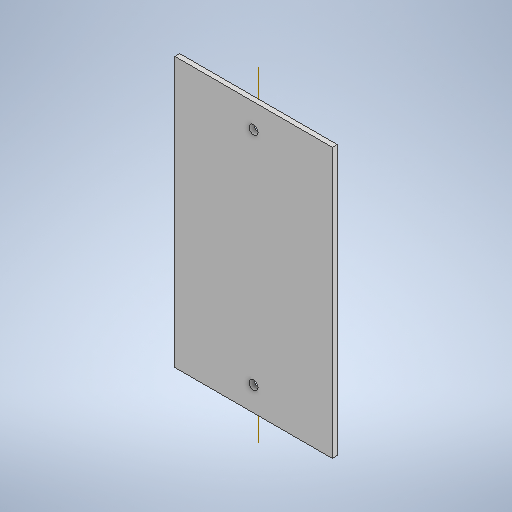
# Autodesk Inventor part: 빵판
Saved by Autodesk Inventor 2025 (Build 290162000, 162)
## iProperties
Created: 2024-06-01
Part Number: 빵판
Material: 일반
Document SubType Name: Modeling
Designer: ckhye
Density: 1 g/cm^3
Appearance: 기본값
Author: ckhye
Autodesk Inventor part; units mm, degrees
ref_plane "YZ Plane" through (0, 0, 0) normal (1, 0, 0) x (0, 1, 0)
ref_plane "XZ Plane" through (0, 0, 0) normal (0, 1, 0) x (-1, 0, 0)
ref_plane "XY Plane" through (0, 0, 0) normal (0, 0, 1) x (1, 0, 0)
sketch "스케치1" plane through (0, 0, 0) normal (0, 0, 1) x (1, 0, 0)
  point P0 (0, 0)
sketch "스케치2" plane through (0, 0, 0) normal (0, 0, 1) x (1, 0, 0)
  line L0 (-26, 44.5) -> (26, 44.5)
  line L1 (26, 44.5) -> (26, -44.5)
  line L2 (26, -44.5) -> (-26, -44.5)
  line L3 (-26, -44.5) -> (-26, 44.5)
  line L4 (-26, 44.5) -> (26, -44.5) construction
  line L5 (26, 44.5) -> (-26, -44.5) construction
  point P0 (0, 0)
  dimension "d0" = 52
  dimension "d1" = 89
  constraints: 12 end point, 2 midpoint, 2 parallel, 1 horizontal, 1 perpendicular
  measures "d0" distance of L1.end L2.end
  measures "d1" distance between parallel lines of L2 L0
extrude "돌출1" add sketch "스케치2" along normal blind 1.6
sketch "스케치3" plane through (0, 0, 1.6) normal (0, 0, 1) x (1, 0, 0)
  circle A0 centre (0, 36.5) radius 1.5
  line L0 (26, 44.5) -> (-26, 44.5) projected
  circle A1 centre (0, -36.5) radius 1.5
  line L1 (-26, -44.5) -> (26, -44.5) projected
  line L2 (0, -62.3) -> (0, 62.3) projected
  point P0 (0, 0)
  dimension "d4" = 3
  dimension "d5" = 8
  dimension "d6" = 3
  dimension "d7" = 8
  constraints: 2 centre point, 2 point on line
  measures "d4" diameter of A0
  measures "d5" distance from line of A0.centre L0
  measures "d6" diameter of A1
  measures "d7" distance from line of L1 A1.centre
extrude "돌출2" cut sketch "스케치3" against normal up to surface (1.6 mm away)
